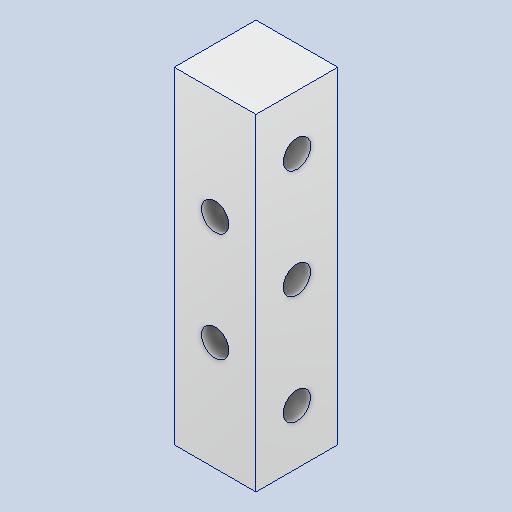
# Autodesk Inventor part: Experimental Block Bracket
Saved by Autodesk Inventor 2023 (Build 270158000, 158)
## iProperties
Created: 2022-08-01
Part Number: Experimental Block Bracket
Material: Aluminum 6061
Document SubType Name: Modeling
Designer: justi
Mass: 66.519 g
Surface Area: 81.1571 cm^2
Volume: 24.6367 cm^3
Density: 2.7 g/cm^3
Appearance: Aluminum - Flat
Author: justi
Autodesk Inventor part; units mm, degrees
ref_plane "YZ Plane" through (0, 0, 0) normal (1, 0, 0) x (0, 1, 0)
ref_plane "XZ Plane" through (0, 0, 0) normal (0, 1, 0) x (-1, 0, 0)
ref_plane "XY Plane" through (0, 0, 0) normal (0, 0, 1) x (1, 0, 0)
sketch "Sketch1" plane through (0, 0, 0) normal (0, 1, 0) x (-1, 0, 0)
  line L0 (0, 0) -> (19.05, 0)
  line L1 (19.05, 0) -> (19.05, -19.05)
  line L2 (19.05, -19.05) -> (0, -19.05)
  line L3 (0, -19.05) -> (0, 0)
  dimension "d0" = 19.05
  dimension "d1" = 19.05
  constraints: 8 end point, 2 parallel, 1 horizontal, 1 perpendicular
  measures "d0" distance of L0.end L1.end
  measures "d1" distance of L1.end L2.end
extrude "Extrusion1" add sketch "Sketch1" along normal blind 76.2
sketch "Sketch4" plane through (-19.05, 0, 0) normal (0, 0, 1) x (1, 0, 0)
  circle A0 centre (9.525, 50.8) radius 3.175
  line L0 (0, 76.2) -> (19.05, 76.2) projected
  line L1 (19.05, 0) -> (19.05, 76.2) projected
  circle A1 centre (9.525, 25.4) radius 3.175
  line L2 (0, 0) -> (19.05, 0) projected
  dimension "d19" = 6.35
  dimension "d20" = 25.4
  dimension "d21" = 9.525
  dimension "d22" = 6.35
  dimension "d23" = 9.525
  dimension "d24" = 25.4
  constraints: 2 centre point
  measures "d19" diameter of A0
  measures "d20" distance from line of L0 A0.centre
  measures "d21" distance from line of L1 A0.centre
  measures "d22" diameter of A1
  measures "d23" distance from line of L1 A1.centre
  measures "d24" distance from line of L2 A1.centre
extrude "Extrusion4" cut sketch "Sketch4" against normal blind 25.4
sketch "Sketch5" plane through (0, 0, 0) normal (1, 0, 0) x (0, 0, -1)
  circle A0 centre (9.5599, 63.5) radius 3.175
  line L0 (0, 76.2) -> (19.05, 76.2) projected
  circle A1 centre (9.525, 38.1) radius 3.175
  line L1 (19.05, 0) -> (19.05, 76.2) projected
  circle A2 centre (9.525, 12.7) radius 3.175
  line L2 (0, 0) -> (19.05, 0) projected
  line L3 (0, 0) -> (0, 76.2) projected
  dimension "d27" = 6.35
  dimension "d28" = 12.7
  dimension "d29" = 6.35
  dimension "d30" = 9.525
  dimension "d31" = 38.1
  dimension "d32" = 6.35
  dimension "d33" = 12.7
  dimension "d34" = 9.525
  constraints: 3 centre point
  measures "d27" diameter of A0
  measures "d28" distance from line of L0 A0.centre
  measures "d29" diameter of A1
  measures "d30" distance from line of L1 A1.centre
  measures "d31" distance from line of L0 A1.centre
  measures "d32" diameter of A2
  measures "d33" distance from line of L2 A2.centre
  measures "d34" distance from line of L3 A2.centre
extrude "Extrusion5" cut sketch "Sketch5" against normal blind 25.4 contours A0 | A1 | A2
body "Solid1"
